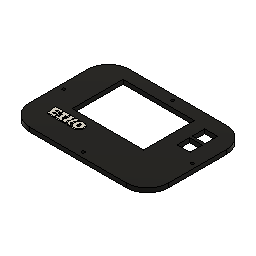
eiko-assembly (Autodesk Fusion 360 archive; units mm, degrees)
design "top plate"
part number: 2026-08-25-02-54-07-841
Autodesk Fusion 360 part; units mm, degrees
note: some values were not read from the file. Chosen so that the rebuilt part matches the saved one: which bodies a step acts on.
sketch "Sketch1" plane through (0, 0, 0) normal (0, 1, 0) x (1, 0, 0)
  line L0 (-1.5154, 62.1887) -> (-1.5154, -12.2213)
  line L1 (-112.7654, -12.2213) -> (-112.7654, 62.1887)
  line L2 (-112.7654, 62.1887) -> (-1.5154, 62.1887)
  line L3 (-1.5154, -12.2213) -> (-112.7654, -12.2213)
  line L4 (-122.7654, 72.1887) -> (8.4846, 72.1887)
  line L5 (-122.7654, -22.2213) -> (-122.7654, 72.1887)
  line L6 (8.4846, 72.1887) -> (8.4846, -22.2213)
  line L7 (8.4846, -22.2213) -> (-122.7654, -22.2213)
  circle A0 centre (-117.7654, 24.9837) radius 1.35
  circle A1 centre (-57.1404, 67.1887) radius 1.35
  circle A2 centre (3.4846, 24.9837) radius 1.35
  circle A3 centre (-57.1404, -17.2213) radius 1.35
sketch "Sketch2" plane through (0, 0, 0) normal (0, 1, 0) x (1, 0, 0)
  line L0 (-106.5854, 60.9687) -> (-21.5854, 60.9687)
  line L1 (-21.5854, 60.9687) -> (-21.5854, 12.9687)
  line L2 (-21.5854, 12.9687) -> (-106.5854, 12.9687)
  line L3 (-106.5854, 12.9687) -> (-106.5854, 60.9687)
  line L4 (-106.5854, 60.9687) -> (-21.5854, 60.9687)
  line L5 (-21.5854, 60.9687) -> (-21.5854, 12.9687)
  line L6 (-21.5854, 12.9687) -> (-106.5854, 12.9687)
  line L7 (-106.5854, 12.9687) -> (-106.5854, 60.9687)
  line L8 (-18.6954, 59) -> (-6.4954, 59)
  line L9 (-6.4954, 59) -> (-6.4954, 47.3)
  line L10 (-6.4954, 47.3) -> (-18.6954, 47.3)
  line L11 (-18.6954, 47.3) -> (-18.6954, 59)
  line L12 (-18.6954, 44.63) -> (-6.4954, 44.63)
  line L13 (-6.4954, 44.63) -> (-6.4954, 32.93)
  line L14 (-6.4954, 32.93) -> (-18.6954, 32.93)
  line L15 (-18.6954, 32.93) -> (-18.6954, 44.63)
  line L16 (-97.8354, 60.9687) -> (-30.3354, 60.9687)
  line L17 (-30.3354, 60.9687) -> (-30.3354, 12.9687)
  line L18 (-30.3354, 12.9687) -> (-97.8354, 12.9687)
  line L19 (-97.8354, 12.9687) -> (-97.8354, 60.9687)
  dimension "d5" = 85
  dimension "d6" = 48
  dimension "d11" = 12.2
  dimension "d12" = 11.7
  dimension "d13" = 2.89
  dimension "d14" = 12.2
  dimension "d15" = 11.7
  dimension "d16" = 2.67
  dimension "d17" = 2.89
  dimension "d28" = 67.5
  dimension "d29" = 8.75
  constraint horizontal L0
  constraint vertical L1
  constraint horizontal L2
  constraint vertical L3
  constraint horizontal L4
  constraint vertical L5
  constraint horizontal L6
  constraint vertical L7
  constraint horizontal L8
  constraint vertical L9
  constraint horizontal L10
  constraint vertical L11
  constraint horizontal L12
  constraint vertical L13
  constraint horizontal L14
  constraint vertical L15
  constraint horizontal L16
  constraint vertical L17
  constraint horizontal L18
  constraint vertical L19
  constraint coincident L4 L16.start
  measures "d5" distance of L0.start L0.end
  measures "d6" distance of L0 L2
  measures "d11" distance of L8.start L8.end
  measures "d12" distance of L8.start L10.end
  measures "d13" distance of L5 L11
  measures "d14" distance of L12.start L12.end
  measures "d15" distance of L12.start L14.end
  measures "d16" distance of L10 L12
  measures "d17" distance of L5 L15
  measures "d28" distance of L16.start L16.end
  measures "d29" distance of L7 L19
extrude "Extrude1" add sketch "Sketch1" along normal blind 4 contours L0 L1 L2 L3 | L4 L5 L6 L7 makes body 1
sketch "Sketch3" plane through (0, 4, 0) normal (0, 1, 0) x (-1, 0, 0)
  circle A0 centre (117.7654, -24.9837) radius 1.35
  circle A1 centre (57.1404, 17.2213) radius 1.35
  circle A2 centre (-3.4846, -24.9837) radius 1.35
  circle A3 centre (57.1404, -67.1887) radius 1.35
  line L0 (-8.4846, 22.2213) -> (-8.4846, -72.1887)
  line L1 (-8.4846, -72.1887) -> (122.7654, -72.1887)
  line L2 (122.7654, -72.1887) -> (122.7654, 22.2213)
  line L3 (122.7654, 22.2213) -> (-8.4846, 22.2213)
extrude "Extrude2" cut sketch "Sketch2" along normal blind 10 bodies 1
fillet "Fillet1" radius 20 4 edges at (-122.7654, 2, 22.2213) (8.4846, 2, 22.2213) (8.4846, 2, -72.1887) (-122.7654, 2, -72.1887) on bodies 1
sketch "Sketch4" plane through (0, 4, 0) normal (0, 1, 0) x (-1, 0, 0)
sketch "Sketch5" plane through (0, 4, 0) normal (0, 1, 0) x (-1, 0, 0)
  line L0 (99.062, -5.8308) -> (106.6622, -5.8308)
  line L1 (106.6622, -5.8308) -> (105.2136, 2.8806)
  line L2 (105.2136, 2.8806) -> (98.804, 2.9004)
  line L3 (98.804, 2.9004) -> (98.804, -0.1357)
  line L4 (98.804, -0.1357) -> (102.8919, 0.8168)
  line L5 (102.8919, 0.8168) -> (102.8919, -0.5325)
  line L6 (102.8919, -0.5325) -> (98.9231, -0.5325)
  line L7 (98.9231, -0.5325) -> (99.062, -2.6955)
  line L8 (99.062, -2.6955) -> (102.8919, -2.4177)
  line L9 (102.8919, -2.4177) -> (102.6934, -3.8068)
  line L10 (102.6934, -3.8068) -> (98.804, -3.1519)
  line L11 (98.804, -3.1519) -> (99.062, -5.8308)
  line L12 (98.2484, 0.539) -> (98.2484, 2.9798)
  line L13 (98.2484, 2.9798) -> (92.5334, 2.8806)
  line L14 (92.5334, 2.8806) -> (92.6922, 0.539)
  line L15 (92.6922, 0.539) -> (94.0217, 0.4795)
  line L16 (94.0217, 0.4795) -> (94.0217, -2.9535)
  line L17 (94.0217, -2.9535) -> (92.5533, -3.1916)
  line L18 (92.5533, -3.1916) -> (92.6922, -6.0491)
  line L19 (92.6922, -6.0491) -> (98.4667, -6.0491)
  line L20 (98.4667, -6.0491) -> (98.4667, -2.5963)
  line L21 (98.4667, -2.5963) -> (96.8792, -2.8543)
  line L22 (96.8792, -2.8543) -> (96.7006, 0.539)
  line L23 (96.7006, 0.539) -> (98.2484, 0.539)
  line L24 (91.819, -6.0094) -> (91.5809, -0.5921)
  line L25 (91.5809, -0.5921) -> (92.0373, -0.5921)
  line L26 (92.0373, -0.5921) -> (92.0373, 2.7417)
  line L27 (92.0373, 2.7417) -> (89.0806, 2.7417)
  line L28 (89.0806, 2.7417) -> (89.0806, -0.5921)
  line L29 (89.0806, -0.5921) -> (86.739, 2.7417)
  line L30 (86.739, 2.7417) -> (84.199, 2.7417)
  line L31 (84.199, 2.7417) -> (86.4612, -0.5921)
  line L32 (86.4612, -0.5921) -> (85.8262, -0.5921)
  line L33 (85.8262, -0.5921) -> (83.6633, -6.0094)
  line L34 (83.6633, -6.0094) -> (87.1161, -6.0094)
  line L35 (87.1161, -6.0094) -> (88.2472, -0.7905)
  line L36 (88.2472, -0.7905) -> (88.2472, -5.8308)
  line L37 (88.2472, -5.8308) -> (91.819, -6.0094)
  line L38 (78.7222, 2.7417) -> (82.4726, 2.7417)
  line L39 (82.4726, 2.7417) -> (84.199, -0.473)
  line L40 (84.199, -0.473) -> (84.199, -3.7671)
  line L41 (84.199, -3.7671) -> (82.4726, -5.9697)
  line L42 (82.4726, -5.9697) -> (78.7222, -5.9697)
  line L43 (78.7222, -5.9697) -> (76.0234, -4.4418)
  line L44 (76.0234, -4.4418) -> (76.0234, 0.162)
  line L45 (76.0234, 0.162) -> (78.7222, 2.7417)
sketch "Sketch6" plane through (0, 4, 0) normal (0, 1, 0) x (-1, 0, 0)
  arc A0 (102.7654, -72.1887) -> (122.7654, -52.1887) centre (102.7654, -52.1887) ccw
  line L0 (122.7654, -52.1887) -> (122.7654, 2.2213)
  arc A1 (122.7654, 2.2213) -> (102.7654, 22.2213) centre (102.7654, 2.2213) ccw
  line L1 (102.7654, 22.2213) -> (11.5154, 22.2213)
  arc A2 (11.5154, 22.2213) -> (-8.4846, 2.2213) centre (11.5154, 2.2213) ccw
  line L2 (-8.4846, 2.2213) -> (-8.4846, -52.1887)
  arc A3 (-8.4846, -52.1887) -> (11.5154, -72.1887) centre (11.5154, -52.1887) ccw
  line L3 (11.5154, -72.1887) -> (102.7654, -72.1887)
  circle A4 centre (57.1404, -67.1887) radius 1.35
  circle A5 centre (-3.4846, -24.9837) radius 1.35
  circle A6 centre (57.1404, 17.2213) radius 1.35
  circle A7 centre (117.7654, -24.9837) radius 1.35
  line L4 (18.6954, -32.93) -> (18.6954, -44.63)
  line L5 (18.6954, -44.63) -> (6.4954, -44.63)
  line L6 (6.4954, -44.63) -> (6.4954, -32.93)
  line L7 (6.4954, -32.93) -> (18.6954, -32.93)
  line L8 (18.6954, -47.3) -> (18.6954, -59)
  line L9 (18.6954, -59) -> (6.4954, -59)
  line L10 (6.4954, -59) -> (6.4954, -47.3)
  line L11 (6.4954, -47.3) -> (18.6954, -47.3)
  line L12 (106.5854, -12.9687) -> (106.5854, -60.9687)
  line L13 (106.5854, -60.9687) -> (21.5854, -60.9687)
  line L14 (21.5854, -60.9687) -> (21.5854, -12.9687)
  line L15 (21.5854, -12.9687) -> (106.5854, -12.9687)
  spline S0 degree 5 poles (81.2674, -1.8727) (81.2639, -1.9898) (81.2506, -2.2237) (81.212, -2.5678) (81.1218, -2.9909) (80.9363, -3.4119) (80.6735, -3.686) (80.3388, -3.7866) (79.9555, -3.7035) (79.5706, -3.4464) (79.2413, -3.0405) (79.0234, -2.5232) (78.9592, -1.9416) (79.0643, -1.349) (79.3168, -0.8028) (79.6717, -0.3579) (80.0714, -0.0622) (80.4582, 0.05) (80.7853, -0.0367) (81.0302, -0.3115) (81.1894, -0.7419) (81.2539, -1.1732) (81.2717, -1.5208) (81.2709, -1.7555) (81.2674, -1.8727) knots 0 0 0 0 0 0 0.05 0.1 0.15 0.2 0.25 0.3 0.35 0.4 0.45 0.5 0.55 0.6 0.65 0.7 0.75 0.8 0.85 0.9 0.95 1 1 1 1 1 1
  point P0 (80.3684, -3.7386)
  point P1 (79, -2)
  point P2 (80.5, 0)
extrude "Extrude3" add sketch "Sketch5" along normal blind 1 separate body makes body 2 at (-89.7156, 4, -4.1441) makes body 3 at (-96.0127, 4, -4.9842) makes body 4 at (-79.6482, 4, -2.0936) makes body 5 at (-104.9225, 4, -1.1609)
extrude "Extrude4" cut sketch "Sketch6" along normal blind 3 contours S0 bodies 4
extrude "Extrude5" add sketch "Sketch2" along normal blind 4 contours L0 L2 L3 L4 L6 L7 L19 bodies 1
extrude "Extrude6" add sketch "Sketch2" along normal blind 4 contours L0 L1 L2 L4 L5 L6 L17 bodies 1

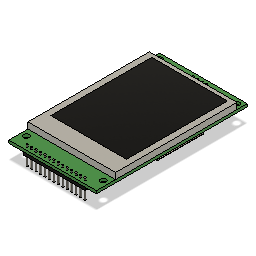
design "_2,8Zoll+TFT+SPI.7f793562-e44e-44ae-986e-20ae59d8bd2c"
Autodesk Fusion 360 part; units mm, degrees
sketch "Skizze1" plane through (0, 0, 0) normal (0, 1, 0) x (1, 0, 0)
  line L0 (0, 0) -> (50, 0)
  line L1 (50, 0) -> (50, 86)
  line L2 (50, 86) -> (0, 86)
  line L3 (0, 86) -> (0, 0)
  circle A0 centre (3, 83) radius 1.6
  circle A1 centre (47, 83) radius 1.6
  circle A2 centre (47, 6.92) radius 1.6
  circle A3 centre (3, 6.92) radius 1.6
  circle A4 centre (8.49, 2) radius 0.5
  circle A5 centre (11.03, 2) radius 0.5
  circle A6 centre (13.57, 2) radius 0.5
  circle A7 centre (16.11, 2) radius 0.5
  circle A8 centre (18.65, 2) radius 0.5
  circle A9 centre (21.19, 2) radius 0.5
  circle A10 centre (23.73, 2) radius 0.5
  circle A11 centre (26.27, 2) radius 0.5
  circle A12 centre (28.81, 2) radius 0.5
  circle A13 centre (31.35, 2) radius 0.5
  circle A14 centre (33.89, 2) radius 0.5
  circle A15 centre (36.43, 2) radius 0.5
  circle A16 centre (38.97, 2) radius 0.5
  circle A17 centre (41.51, 2) radius 0.5
  line L4 (25, 86) -> (25, 0) construction
  line L5 (0, 84) -> (50, 84) construction
  circle A18 centre (23.73, 84) radius 0.5
  circle A19 centre (26.27, 84) radius 0.5
  circle A20 centre (28.81, 84) radius 0.5
  circle A21 centre (21.19, 84) radius 0.5
  dimension "d1" = 50
  dimension "d2" = 86
  dimension "d3" = 3.2
  dimension "d4" = 3.2
  dimension "d5" = 3.2
  dimension "d6" = 3.2
  dimension "d7" = 6.92
  dimension "d8" = 6.92
  dimension "d9" = 3
  dimension "d10" = 3
  dimension "d11" = 3
  dimension "d12" = 3
  dimension "d13" = 3
  dimension "d14" = 3
  dimension "d15" = 1
  dimension "d16" = 8.49
  dimension "d17" = 2
  dimension "d20" = 2.54
  dimension "d21" = 0
  dimension "d22" = 8.49
  dimension "d36" = 2
  dimension "d37" = 1
  dimension "d38" = 1
  dimension "d39" = 1
  dimension "d40" = 1
  dimension "d41" = 1.27
  dimension "d42" = 1.27
  dimension "d43" = 2.54
  dimension "d44" = 2.54
  measures "d3" diameter of A0
  measures "d4" diameter of A1
  measures "d5" diameter of A2
  measures "d6" diameter of A3
  measures "d15" diameter of A4
  measures "d36" distance of L2 L5
  measures "d37" diameter of A18
  measures "d38" diameter of A19
  measures "d39" diameter of A20
  measures "d40" diameter of A21
extrude "Extrusion1" add sketch "Skizze1" along normal blind 1.6 makes body 1
sketch "Skizze2" plane through (0, 1.6, 0) normal (0, 1, 0) x (-1, 0, 0)
  circle A0 centre (-16.11, -2) radius 0.5
  circle A1 centre (-18.65, -2) radius 0.5
  circle A2 centre (-21.19, -2) radius 0.5
  circle A3 centre (-23.73, -2) radius 0.5
  circle A4 centre (-26.27, -2) radius 0.5
  circle A5 centre (-13.57, -2) radius 0.5
  circle A6 centre (-11.03, -2) radius 0.5
  circle A7 centre (-8.49, -2) radius 0.5
  circle A8 centre (-3, -6.92) radius 1.6
  circle A9 centre (-47, -6.92) radius 1.6
  circle A10 centre (-47, -83) radius 1.6
  circle A11 centre (-3, -83) radius 1.6
  circle A12 centre (-28.81, -2) radius 0.5
  circle A13 centre (-33.89, -2) radius 0.5
  circle A14 centre (-36.43, -2) radius 0.5
  circle A15 centre (-38.97, -2) radius 0.5
  circle A16 centre (-41.51, -2) radius 0.5
  circle A17 centre (-31.35, -2) radius 0.5
  line L0 (0, -86) -> (0, 0)
  line L1 (0, 0) -> (-50, 0)
  line L2 (-50, 0) -> (-50, -86)
  line L3 (-50, -86) -> (0, -86)
  line L4 (0, -80.2) -> (-50, -80.2)
  line L5 (-50, -80.2) -> (-50, -10.9)
  line L6 (-50, -10.9) -> (0, -10.9)
  line L7 (0, -10.9) -> (0, -80.2)
  circle A18 centre (-28.81, -84) radius 0.5
  circle A19 centre (-23.73, -84) radius 0.5
  circle A20 centre (-26.27, -84) radius 0.5
  circle A21 centre (-21.19, -84) radius 0.5
  dimension "d25" = 5.8
  dimension "d26" = 10.9
  measures "d25" distance of L3 L4
  measures "d26" distance of L1 L6
extrude "Extrusion2" add sketch "Skizze2" along normal blind 3.54 separate body contours L0 L2 L4 L5 L6 L7 makes body 2
sketch "Skizze3" plane through (0, 5.14, 0) normal (0, 1, 0) x (-1, 0, 0)
  line L0 (0, -10.9) -> (-50, -10.9)
  line L1 (-50, -10.9) -> (-50, -80.2)
  line L2 (-50, -80.2) -> (0, -80.2)
  line L3 (0, -80.2) -> (0, -10.9)
  line L4 (-3.4, -78.15) -> (-46.6, -78.15)
  line L5 (-46.6, -78.15) -> (-46.6, -20.55)
  line L6 (-46.6, -20.55) -> (-3.4, -20.55)
  line L7 (-3.4, -20.55) -> (-3.4, -78.15)
  line L8 (-25, -80.2) -> (-25, -10.9) construction
  dimension "d29" = 43.2
  dimension "d30" = 57.6
  dimension "d31" = 21.6
  dimension "d32" = 2.05
  dimension "d33" = 3.4
  measures "d29" distance of origin
  measures "d30" distance of L4 L6
  measures "d31" distance of L7 L8
  measures "d32" distance of L2 L4
  measures "d33" distance of L1 L5
extrude "Extrusion3" cut sketch "Skizze3" against normal blind 0.01 contours L4 L5 L6 L7 bodies 2
sketch "Skizze4" plane through (0, 0, 0) normal (0, -1, 0) x (1, 0, 0)
  circle A0 centre (28.81, -84) radius 0.5
  circle A1 centre (41.51, -2) radius 0.5
  circle A2 centre (23.73, -84) radius 0.5
  circle A3 centre (26.27, -84) radius 0.5
  circle A4 centre (23.73, -2) radius 0.5
  circle A5 centre (21.19, -84) radius 0.5
  circle A6 centre (26.27, -2) radius 0.5
  circle A7 centre (28.81, -2) radius 0.5
  circle A8 centre (31.35, -2) radius 0.5
  circle A9 centre (33.89, -2) radius 0.5
  circle A10 centre (36.43, -2) radius 0.5
  circle A11 centre (38.97, -2) radius 0.5
  circle A12 centre (21.19, -2) radius 0.5
  circle A13 centre (18.65, -2) radius 0.5
  circle A14 centre (16.11, -2) radius 0.5
  circle A15 centre (13.57, -2) radius 0.5
  circle A16 centre (11.03, -2) radius 0.5
  circle A17 centre (8.49, -2) radius 0.5
  circle A18 centre (3, -6.92) radius 1.6
  circle A19 centre (47, -6.92) radius 1.6
  circle A20 centre (47, -83) radius 1.6
  circle A21 centre (3, -83) radius 1.6
  line L0 (0, 0) -> (0, -86)
  line L1 (0, -86) -> (50, -86)
  line L2 (50, -86) -> (50, 0)
  line L3 (50, 0) -> (0, 0)
  line L4 (31.4, -36.8) -> (48, -36.8)
  line L5 (48, -36.8) -> (48, -63.3)
  line L6 (48, -63.3) -> (31.4, -63.3)
  line L7 (31.4, -63.3) -> (31.4, -36.8)
  dimension "d45" = 16.6
  dimension "d46" = 2
  dimension "d47" = 36.8
  dimension "d48" = 22.7
  measures "d45" distance of L5 L7
  measures "d46" distance of L2 L5
  measures "d47" distance of L3 L4
  measures "d48" distance of L1 L6
extrude "Extrusion4" add sketch "Skizze4" along normal blind 2.95 separate body contours L4 L5 L6 L7 makes body 3
sketch "Skizze5" plane through (48, 0, 0) normal (1, 0, 0) x (0, 0, -1)
  line L0 (63.3, 0) -> (36.8, 0)
  line L1 (36.8, 0) -> (36.8, -2.95)
  line L2 (36.8, -2.95) -> (63.3, -2.95)
  line L3 (63.3, -2.95) -> (63.3, 0)
  line L4 (38, -0.25) -> (62.1, -0.25)
  line L5 (62.1, -0.25) -> (62.1, -2.75)
  line L6 (62.1, -2.75) -> (38, -2.75)
  line L7 (38, -2.75) -> (38, -0.25)
  dimension "d51" = 0.2
  dimension "d52" = 1.2
  dimension "d53" = 1.2
  dimension "d54" = 2.5
  measures "d51" distance of L2 L6
  measures "d52" distance of L3 L5
  measures "d53" distance of L1 L7
  measures "d54" distance of L4 L6
extrude "Extrusion5" cut sketch "Skizze5" against normal blind 15 contours L4 L5 L6 L7 bodies 3
sketch "Skizze6" plane through (0, 0, 0) normal (0, -1, 0) x (1, 0, 0)
  circle A0 centre (28.81, -84) radius 0.5
  circle A1 centre (41.51, -2) radius 0.5
  circle A2 centre (23.73, -84) radius 0.5
  circle A3 centre (26.27, -84) radius 0.5
  circle A4 centre (23.73, -2) radius 0.5
  circle A5 centre (21.19, -84) radius 0.5
  circle A6 centre (26.27, -2) radius 0.5
  circle A7 centre (28.81, -2) radius 0.5
  circle A8 centre (31.35, -2) radius 0.5
  circle A9 centre (33.89, -2) radius 0.5
  circle A10 centre (36.43, -2) radius 0.5
  circle A11 centre (38.97, -2) radius 0.5
  circle A12 centre (21.19, -2) radius 0.5
  circle A13 centre (18.65, -2) radius 0.5
  circle A14 centre (16.11, -2) radius 0.5
  circle A15 centre (13.57, -2) radius 0.5
  circle A16 centre (11.03, -2) radius 0.5
  circle A17 centre (8.49, -2) radius 0.5
  circle A18 centre (3, -6.92) radius 1.6
  circle A19 centre (47, -6.92) radius 1.6
  circle A20 centre (47, -83) radius 1.6
  circle A21 centre (3, -83) radius 1.6
  line L0 (0, 0) -> (0, -86)
  line L1 (0, -86) -> (50, -86)
  line L2 (50, -86) -> (50, 0)
  line L3 (50, 0) -> (0, 0)
  circle A22 centre (8.49, -2) radius 0.5
  circle A23 centre (11.03, -2) radius 0.5
  circle A24 centre (13.57, -2) radius 0.5
  circle A25 centre (16.11, -2) radius 0.5
  circle A26 centre (18.65, -2) radius 0.5
  circle A27 centre (21.19, -2) radius 0.5
  circle A28 centre (23.73, -2) radius 0.5
  circle A29 centre (26.27, -2) radius 0.5
  circle A30 centre (28.81, -2) radius 0.5
  circle A31 centre (31.35, -2) radius 0.5
  circle A32 centre (33.89, -2) radius 0.5
  circle A33 centre (36.43, -2) radius 0.5
  circle A34 centre (38.97, -2) radius 0.5
  circle A35 centre (41.51, -2) radius 0.5
extrude "Extrusion6" add sketch "Skizze6" along normal blind 8 and the other way blind 2.8 separate body contours A1 A35 | A4 A28 | A6 A29 | A7 A30 | A8 A31 | A9 A32 | A10 A33 | A11 A34 | A12 A27 | A13 A26 | A14 A25 | A15 A24 | A16 A23 | A17 A22 makes body 4 at (36.0809, -5.3333, -1.6421) makes body 5 at (26.4054, -5.3333, -1.5187) makes body 6 at (16.4408, -2.6667, -2.3749) makes body 7 at (8.9894, -5.3333, -2.0249) makes body 8 at (18.3009, -5.3333, -1.6421) makes body 9 at (28.9454, -5.3333, -1.5187) makes body 10 at (38.6209, -5.3333, -1.6421) makes body 11 at (33.5409, -5.3333, -1.6421) makes body 12 at (23.8654, -5.3333, -1.5187) makes body 13 at (14.0694, -5.3333, -2.0249) makes body 14 at (11.5294, -5.3333, -2.0249) makes body 15 at (21.3254, -5.3333, -1.5187) makes body 16 at (31.8494, -5.3333, -2.0249) makes body 17 at (41.1609, -5.3333, -1.6421)
sketch "Skizze7" plane through (0, 0, 0) normal (0, -1, 0) x (1, 0, 0)
  circle A0 centre (28.81, -84) radius 0.5
  circle A1 centre (41.51, -2) radius 0.5
  circle A2 centre (23.73, -84) radius 0.5
  circle A3 centre (26.27, -84) radius 0.5
  circle A4 centre (23.73, -2) radius 0.5
  circle A5 centre (21.19, -84) radius 0.5
  circle A6 centre (26.27, -2) radius 0.5
  circle A7 centre (28.81, -2) radius 0.5
  circle A8 centre (31.35, -2) radius 0.5
  circle A9 centre (33.89, -2) radius 0.5
  circle A10 centre (36.43, -2) radius 0.5
  circle A11 centre (38.97, -2) radius 0.5
  circle A12 centre (21.19, -2) radius 0.5
  circle A13 centre (18.65, -2) radius 0.5
  circle A14 centre (16.11, -2) radius 0.5
  circle A15 centre (13.57, -2) radius 0.5
  circle A16 centre (11.03, -2) radius 0.5
  circle A17 centre (8.49, -2) radius 0.5
  circle A18 centre (3, -6.92) radius 1.6
  circle A19 centre (47, -6.92) radius 1.6
  circle A20 centre (47, -83) radius 1.6
  circle A21 centre (3, -83) radius 1.6
  line L0 (0, 0) -> (0, -86)
  line L1 (0, -86) -> (50, -86)
  line L2 (50, -86) -> (50, 0)
  line L3 (50, 0) -> (0, 0)
  line L4 (7.29, -0.8) -> (42.71, -0.8)
  line L5 (42.71, -0.8) -> (42.71, -3.2)
  line L6 (42.71, -3.2) -> (7.29, -3.2)
  line L7 (7.29, -3.2) -> (7.29, -0.8)
  dimension "d59" = 1.2
  dimension "d60" = 1.2
  dimension "d61" = 1.2
  dimension "d62" = 1.2
  measures "d59" distance of L4
  measures "d60" distance of L6
  measures "d61" distance of L7
  measures "d62" distance of L5
extrude "Extrusion7" add sketch "Skizze7" along normal blind 2.4 separate body contours L4 L5 L6 L7 makes body 18
equation "d31 = ( 43.2 / 2 ) * 1 mm"
